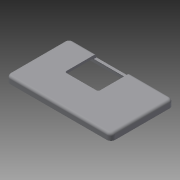
# Autodesk Inventor part: Beta_V2_Top01
Saved by Autodesk Inventor 2013 (Build 170138000, 138)
## iProperties
Created: 2015-02-17
Part Number: Beta_V2_Top01
Material: Generic
Document SubType Name: Modeling
Designer: spichelh
Density: 1 g/cm^3
Author: spichelh
Autodesk Inventor part; units mm, degrees
ref_plane "YZ Plane" through (0, 0, 0) normal (1, 0, 0) x (0, 1, 0)
ref_plane "XZ Plane" through (0, 0, 0) normal (0, 1, 0) x (-1, 0, 0)
ref_plane "XY Plane" through (0, 0, 0) normal (0, 0, 1) x (1, 0, 0)
sketch "Sketch1" plane through (0, 0, 0) normal (0, 1, 0) x (-1, 0, 0)
  line L0 (57.5, -65) -> (-57.5, -65)
  line L1 (-62.5, -60) -> (-62.5, 5)
  line L2 (-57.5, 10) -> (57.5, 10)
  line L3 (62.5, 5) -> (62.5, -60)
  arc A0 (-57.5, 10) -> (-62.5, 5) centre (-57.5, 5) ccw
  arc A1 (62.5, 5) -> (57.5, 10) centre (57.5, 5) ccw
  arc A2 (57.5, -65) -> (62.5, -60) centre (57.5, -60) ccw
  arc A3 (-62.5, -60) -> (-57.5, -65) centre (-57.5, -60) ccw
  line L4 (0, 10) -> (0, -20.4446) construction
  point P0 (0, 0)
  point P1 (62.5, -65)
  point P2 (-62.5, 10)
  point P3 (62.5, 10)
  dimension "d0" = 125
  dimension "d4" = 75
  dimension "d5" = 5
  dimension "d9" = 10
  constraints: 10 end point, 8 point on circle, 8 tangent, 7 point on line, 4 centre point, 3 equal radius, 3 parallel, 1 horizontal, 1 midpoint, 1 perpendicular
  measures "d0" distance of point (-62.5, 10) point (62.5, 10)
  measures "d4" distance of point (62.5, 10) point (62.5, -65)
  measures "d5" radius of A0
  measures "d9" distance from line of L2 point (0, 0)
extrude "Extrusion1" add sketch "Sketch1" along normal blind 8
fillet "Fillet1" radius 3 8 edges at (-61.0355, 8, 8.5355) (0, 8, 10) (61.0355, 8, 8.5355) (62.5, 8, -27.5) (61.0355, 8, -63.5355) (0, 8, -65) (-61.0355, 8, -63.5355) (-62.5, 8, -27.5)
sketch "Sketch2" plane through (0, 0, 0) normal (0, -1, 0) x (1, 0, 0)
  line L0 (62.5, 5) -> (62.5, -60) projected
  arc A0 (62.5, 5) -> (57.5, 10) centre (57.5, 5) ccw projected
  line L1 (-57.5, 10) -> (57.5, 10) projected
  arc A1 (-57.5, 10) -> (-62.5, 5) centre (-57.5, 5) ccw projected
  line L2 (-62.5, -60) -> (-62.5, 5) projected
  arc A2 (-62.5, -60) -> (-57.5, -65) centre (-57.5, -60) ccw projected
  line L3 (57.5, -65) -> (-57.5, -65) projected
  arc A3 (57.5, -65) -> (62.5, -60) centre (57.5, -60) ccw projected
  arc A4 (59.5, 5) -> (57.5, 7) centre (57.5, 5) ccw
  line L4 (59.5, 5) -> (59.5, -60)
  arc A5 (57.5, -62) -> (59.5, -60) centre (57.5, -60) ccw
  line L5 (57.5, -62) -> (-57.5, -62)
  arc A6 (-59.5, -60) -> (-57.5, -62) centre (-57.5, -60) ccw
  line L6 (-59.5, -60) -> (-59.5, 5)
  arc A7 (-57.5, 7) -> (-59.5, 5) centre (-57.5, 5) ccw
  line L7 (-57.5, 7) -> (57.5, 7)
  point P0 (0, 0)
  dimension "d10" = 3
  constraints: 8 end point, 8 point on circle, 4 centre point, 7 other
  measures "d10" distance between parallel lines of L1 L7
extrude "Extrusion2" cut sketch "Sketch2" against normal blind 5 contours L4 A5 L5 A6 L6 A7 L7 A4
fillet "Fillet2" radius 2 8 edges at (-58.9142, 5, -61.4142) (-59.5, 5, -27.5) (-58.9142, 5, 6.4142) (0, 5, 7) (58.9142, 5, 6.4142) (59.5, 5, -27.5) (58.9142, 5, -61.4142) (0, 5, -62)
sketch "Sketch3" plane through (0, 8, 0) normal (0, 1, 0) x (1, 0, 0)
  line L0 (-57.5, 62) -> (57.5, 62) projected
  line L1 (-27.7, 67) -> (8.3, 67)
  line L2 (10.3, 65) -> (10.3, 29)
  line L3 (8.3, 27) -> (-27.7, 27)
  line L4 (-29.7, 29) -> (-29.7, 65)
  arc A0 (-27.7, 67) -> (-29.7, 65) centre (-27.7, 65) ccw
  arc A1 (10.3, 65) -> (8.3, 67) centre (8.3, 65) ccw
  arc A2 (8.3, 27) -> (10.3, 29) centre (8.3, 29) ccw
  arc A3 (-29.7, 29) -> (-27.7, 27) centre (-27.7, 29) ccw
  line L5 (62.5, -5) -> (62.5, 60) projected
  line L6 (-62.5, 60) -> (-62.5, -5) projected
  point P0 (0, 0)
  point P1 (10.3, 27)
  point P2 (10.3, 67)
  point P3 (-29.7, 27)
  point P4 (-9.7, 67)
  dimension "d14" = 40
  dimension "d15" = 40
  dimension "d16" = 2
  dimension "d17" = 5
  dimension "d21" = 52.8
  constraints: 8 end point, 8 point on circle, 8 tangent, 6 point on line, 4 centre point, 3 equal radius, 2 parallel, 1 horizontal, 1 midpoint, 1 perpendicular
  measures "d14" distance of point (10.3, 27) point (-29.7, 27)
  measures "d15" distance of point (10.3, 67) point (10.3, 27)
  measures "d16" radius of A0
  measures "d17" distance between parallel lines of L1 L0
  measures "d21" distance from line of L6 point (-9.7, 67)
extrude "Extrusion3" cut sketch "Sketch3" against normal blind 4
body "Solid1"
